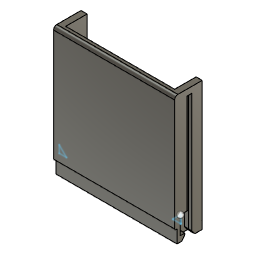
ExpansionCard (Autodesk Fusion 360 design; units mm, degrees)
Autodesk Fusion 360 part; units mm, degrees
sketch "Sketch1" plane through (0, 0, 0) normal (0, 0, 1) x (1, 0, 0)
ref_plane "WorkPlane1" through (0, 0, 0) normal (0, 0, 1) x (1, 0, 0)
sketch "Sketch2" plane through (0, 0, 0) normal (0, 0, 1) x (1, 0, 0)
  line L0 (-0.0018, 6.8149) -> (30, 6.8149)
  line L1 (30, 6.8149) -> (30, 0)
  line L2 (30, 0) -> (-0.0018, 0)
  line L3 (-0.0018, 0) -> (-0.0018, 6.8149)
  line L4 (14.9991, 3.4075) -> (25.7991, 3.4075)
  line L5 (14.9991, 3.4075) -> (4.1991, 3.4075)
  line L6 (14.9991, 4.3075) -> (4.6991, 4.3075)
  line L7 (14.9991, 4.3075) -> (25.2991, 4.3075)
  line L8 (14.9991, 2.5075) -> (4.6991, 2.5075)
  line L9 (14.9991, 2.5075) -> (25.2991, 2.5075)
  line L10 (14.9991, 4.3075) -> (25.2991, 4.3075)
  line L11 (14.9991, 4.3075) -> (4.6991, 4.3075)
  line L12 (25.7991, 3.8075) -> (25.7991, 3.4075)
  line L13 (4.1991, 3.0075) -> (4.1991, 3.4075)
  line L14 (4.1991, 3.8075) -> (4.1991, 3.4075)
  line L15 (25.7991, 3.4075) -> (25.7991, 3.0075)
  arc A0 (4.6991, 4.3075) -> (4.1991, 3.8075) centre (4.6991, 3.8075) ccw
  arc A1 (4.1991, 3.0075) -> (4.6991, 2.5075) centre (4.6991, 3.0075) ccw
  arc A2 (25.2991, 2.5075) -> (25.7991, 3.0075) centre (25.2991, 3.0075) ccw
  arc A3 (25.7991, 3.8075) -> (25.2991, 4.3075) centre (25.2991, 3.8075) ccw
  line L16 (14.9991, 3.4075) -> (14.9995, 3.4074)
  line L17 (15, 3.4075) -> (14.9995, 3.4074)
  dimension "d2" = 10.8
  dimension "d3" = 10.8
  dimension "d8" = 0.5
  constraint horizontal L0
  constraint vertical L1
  constraint horizontal L2
  constraint vertical L3
  constraint parallel L2 L4
  constraint parallel L4 L5
  constraint perpendicular L4 L12
  constraint perpendicular L5 L13
  constraint perpendicular L5 L14
  constraint parallel L5 L6
  constraint parallel L4 L7
  constraint tangent L14 A0
  constraint tangent L6 A0
  constraint parallel L5 L8
  constraint tangent L13 A1
  constraint tangent L8 A1
  constraint equal A0 A1
  constraint parallel L4 L9
  constraint tangent L9 A2
  constraint tangent L15 A2
  constraint equal A0 A2
  constraint tangent L12 A3
  constraint tangent L7 A3
  constraint equal A0 A3
  constraint parallel L4 L10
  constraint parallel L5 L11
  constraint coincident L4 L17.start
  measures "d2" distance of L4.start L4.end
  measures "d3" distance of L4.start L5.end
  measures "d8" radius of A0
other "Base Mesh Feature2"
sketch "Sketch4" plane through (0, 0, 0) normal (1, 0, 0) x (0, 1, 0)
  line L0 (6.8002, -0.0004) -> (6.8002, 32)
  line L1 (6.8002, 32) -> (0.8415, 32)
  line L2 (6.8002, -0.0004) -> (-0.2407, -0.0004)
  line L3 (-0.0066, 3.4989) -> (-0.0585, 31.0983)
  line L4 (4.9902, -0.0004) -> (4.2999, 0.9325)
  line L5 (4.2999, 0.9325) -> (4.25, 0.9325)
  line L6 (4.25, 0.9325) -> (4.25, 4.0597)
  line L7 (4.25, 4.0597) -> (2.5001, 4.0597)
  line L8 (2.5001, 1.39) -> (2.5001, 0.9325)
  line L9 (2.5001, 0.9325) -> (2.4506, 0.9325)
  line L10 (2.4506, 0.9325) -> (1.7589, -0.0004)
  line L11 (2.5001, 1.39) -> (1.4001, 1.39)
  line L12 (1.4001, 1.39) -> (1.4001, 5.86)
  line L13 (1.4001, 5.86) -> (3.0784, 5.86)
  line L14 (3.0784, 5.86) -> (3.0784, 30.5)
  line L15 (3.0784, 30.5) -> (4.25, 30.5)
  line L16 (4.25, 30.5) -> (4.25, 4.0597)
  line L17 (0.5999, -0.0004) -> (0.5999, 3.2)
  line L18 (0.5999, 3.2) -> (0.294, 3.1994)
  arc A0 (0.8415, 32) -> (-0.0585, 31.0983) centre (0.8415, 31.1) ccw
  arc A1 (-0.0066, 3.4989) -> (0.294, 3.1994) centre (0.2934, 3.4994) ccw
  line L19 (2.5001, 4.0597) -> (1.4001, 4.0597)
  dimension "d9" = 0.9
  dimension "d10" = 0.3
  constraint vertical L0
  constraint perpendicular L0 L1
  constraint perpendicular L0 L2
  constraint coincident L2 L4.start
  constraint parallel L2 L5
  constraint perpendicular L5 L6
  constraint perpendicular L6 L7
  constraint perpendicular L7 L8
  constraint perpendicular L8 L9
  constraint coincident L2 L10.end
  constraint perpendicular L8 L11
  constraint perpendicular L11 L12
  constraint perpendicular L12 L13
  constraint perpendicular L13 L14
  constraint perpendicular L14 L15
  constraint coincident L2 L17.start
  constraint perpendicular L2 L17
  constraint perpendicular L3 L18
  constraint tangent L1 A0
  constraint tangent L3 A0
  constraint tangent L18 A1
  constraint tangent L3 A1
  constraint coincident L12 L19.end
  constraint perpendicular L12 L19
  measures "d9" radius of A0
  measures "d10" radius of A1
ref_plane "WorkPlane2" through (14.9991, 3.4075, 32) normal (0, 0, 1) x (1, 0, 0)
sketch "Sketch5" plane through (14.9991, 3.4075, 32) normal (0, 0, 1) x (1, 0, 0)
  line L0 (-14.9991, 3.3927) -> (-14.9991, -3.4075)
  line L1 (-14.9991, -3.4075) -> (15.0009, -3.4075)
  line L2 (15.0009, -3.4075) -> (15.0009, 3.4075)
  line L3 (13.5009, 3.3927) -> (13.5009, 3.4067)
  line L4 (13.5009, 3.3927) -> (13.5009, -1.9074)
  line L5 (13.5009, -1.9074) -> (-13.4991, -1.9074)
  line L6 (-13.4991, -1.9074) -> (-13.5017, 3.3934)
  line L7 (15.0009, 3.4075) -> (13.5009, 3.4067)
  line L8 (-13.5017, 3.3934) -> (-14.9991, 3.3927)
  point P0 (-14.9991, 3.3927)
  point P1 (-14.9991, -3.4075)
  point P2 (15.0009, -3.4075)
  point P3 (15.0009, 3.4075)
  constraint coincident P0 L0.start
  constraint coincident P1 L0.end
  constraint coincident P2 L1.end
  constraint coincident P3 L2.end
  constraint perpendicular L3 L7
  constraint perpendicular L1 L4
  constraint perpendicular L4 L5
  constraint coincident L6.end L7
  constraint perpendicular L6 L7
  constraint collinear L7 L8
other "Modify1"
extrude "Extrude1" add sketch "Sketch5" against normal blind 32
extrude "Extrude2" add sketch "Sketch2" along normal blind 2
other "Modify2"
sketch "Side Slats" plane through (0, 0, 0) normal (0, 0, 1) x (1, 0, 0)
  line L0 (29.9999, 3.0777) -> (29.19, 3.93)
  line L1 (29.19, 3.93) -> (29.19, 4.25)
  line L2 (29.19, 4.25) -> (30, 4.25)
  line L3 (-0.0001, 3.0776) -> (0.81, 3.93)
  line L4 (0.81, 3.93) -> (0.81, 4.25)
  line L5 (0.81, 4.25) -> (0, 4.25)
  line L6 (-0.0001, 3.0776) -> (-0.201, 2.8662)
  line L7 (-0.201, 2.8662) -> (-0.2009, 4.25)
  line L8 (0, 4.25) -> (-0.2009, 4.25)
  line L9 (30, 4.25) -> (30.168, 4.25)
  line L10 (29.9999, 3.0777) -> (30.168, 2.9008)
  line L11 (30.168, 2.9008) -> (30.168, 4.25)
  constraint vertical L1
  constraint perpendicular L1 L2
  constraint vertical L4
  constraint perpendicular L4 L5
  constraint parallel L3 L6
  constraint perpendicular L7 L8
  constraint parallel L0 L10
  constraint perpendicular L9 L11
extrude "Extrude16" cut sketch "Side Slats" along normal blind 30.5
sketch "Sketch7" plane through (0, 0, 0) normal (1, 0, 0) x (0, 1, 0)
extrude "Extrude4" cut sketch "Sketch4" along normal blind 1.8 contours L2 L4 L5 L6 L7 L8 L9 L10 L11 L12 L19
extrude "Extrude5" cut sketch "Sketch4" against normal blind 1.2 contours L2 L4 L5 L6 L7 L8 L9 L10 L11 L12 L19
ref_plane "WorkPlane3" through (30, 0, 0) normal (1, 0, 0) x (0, 1, 0)
sketch "Sketch8" plane through (30, 0, 0) normal (1, 0, 0) x (0, 1, 0)
  line L0 (1.76, 0) -> (2.4501, 0.9324)
  line L1 (2.4501, 0.9324) -> (2.5001, 0.9324)
  line L2 (2.5001, 0.9324) -> (2.5001, 1.3897)
  line L3 (2.5001, 4.0595) -> (4.25, 4.0602)
  line L4 (4.25, 4.0602) -> (4.25, 0.9324)
  line L5 (4.25, 0.9324) -> (4.3, 0.9324)
  line L6 (4.3, 0.9324) -> (4.9902, -0.0001)
  line L7 (4.9902, -0.0001) -> (1.76, 0)
  line L8 (2.5001, 1.3897) -> (1.4001, 1.3897)
  line L9 (1.4001, 1.3897) -> (1.4001, 4.06)
  line L10 (1.4001, 4.06) -> (2.5001, 4.0595)
  constraint horizontal L1
  constraint perpendicular L1 L2
  constraint perpendicular L1 L4
  constraint perpendicular L4 L5
  constraint perpendicular L2 L8
  constraint perpendicular L8 L9
extrude "Extrude6" cut sketch "Sketch8" against normal blind 1.8
ref_plane "WorkPlane4" through (0, 0, 1.5) normal (0, 0, 1) x (1, 0, 0)
sketch "Sketch9" plane through (0, 0, 1.5) normal (0, 0, 1) x (1, 0, 0)
  line L0 (1.5, 5.3) -> (2.5, 5.3)
  line L1 (2.5, 5.3) -> (2.5, 1.5)
  line L2 (2.5, 1.5) -> (1.5, 1.5)
  line L3 (28.5, 5.3) -> (27.5, 5.3)
  line L4 (27.5, 5.3) -> (27.5, 1.5001)
  line L5 (27.5, 1.5001) -> (28.5, 1.5001)
  line L6 (1.6305, 5.3) -> (1.4386, 5.3)
  line L7 (1.4386, 5.3) -> (1.4386, 1.5)
  line L8 (1.4386, 1.5) -> (1.5958, 1.5)
  line L9 (28.4487, 5.3) -> (28.5452, 5.3)
  line L10 (28.5452, 5.3) -> (28.5453, 1.5001)
  line L11 (28.4238, 1.5001) -> (28.5453, 1.5001)
  constraint horizontal L0
  constraint perpendicular L0 L1
  constraint perpendicular L1 L2
  constraint horizontal L3
  constraint perpendicular L3 L4
  constraint perpendicular L4 L5
  constraint coincident L0 L6.start
  constraint parallel L0 L6
  constraint perpendicular L2 L7
  constraint coincident L2 L8.end
  constraint parallel L2 L8
  constraint coincident L3 L9.start
  constraint perpendicular L9 L10
  constraint coincident L5 L11.start
  constraint perpendicular L10 L11
extrude "Extrude7" add sketch "Sketch9" along normal blind 4 contours L0 L1 L2 L6 L7 L8
extrude "Extrude8" add sketch "Sketch9" along normal blind 4 contours L3 L4 L5 L9 L10 L11
ref_plane "WorkPlane5" through (0, 6, 0) normal (0, 1, 0) x (0, 0, 1)
sketch "Sketch10" plane through (0, 6, 0) normal (0, 1, 0) x (1, 0, 0)
  line L0 (2.5, -4.5) -> (1.5001, -5.5)
  line L1 (1.5001, -5.5) -> (2.5, -5.5)
  line L2 (2.5, -5.5) -> (2.5, -4.5)
  line L3 (28.5, -5.5) -> (27.5, -5.5)
  line L4 (27.5, -5.5) -> (27.5, -4.5)
  line L5 (27.5, -4.5) -> (28.5, -5.5)
  constraint horizontal L1
  constraint perpendicular L1 L2
  constraint perpendicular L2 L3
  constraint perpendicular L3 L4
extrude "Extrude9" cut sketch "Sketch10" against normal blind 4.5
extrude "Extrude10" cut sketch "Sketch8" against normal blind 1.8
extrude "Extrude11" cut sketch "Sketch4" along normal blind 1.8 contours L2 L4 L5 L6 L7 L8 L9 L10 L11 L12 L19
sketch "Sketch11" plane through (30, 0, 0) normal (1, 0, 0) x (0, 1, 0)
  line L0 (1.76, 0) -> (2.4501, 0.9324)
  line L1 (2.4501, 0.9324) -> (2.5001, 0.9324)
  line L2 (2.5001, 0.9324) -> (2.5001, 1.3897)
  line L3 (2.5001, 1.3897) -> (1.4001, 1.3897)
  line L4 (1.4001, 1.3897) -> (1.4001, 4.06)
  line L5 (1.4001, 4.06) -> (2.5001, 4.0595)
  line L6 (2.5001, 4.0595) -> (3.0776, 4.0597)
  line L7 (6.8149, 32) -> (0, 32)
  line L8 (0, 32) -> (0, 0)
  line L9 (4.9901, 0) -> (6.8149, 0)
  line L10 (0.6001, 0) -> (0.012, 0)
  line L11 (0.012, 3.1995) -> (0.6001, 3.1995)
  line L12 (0.6001, 3.1995) -> (0.6001, 0)
  line L13 (0.0679, 0) -> (-0.3097, 0)
  line L14 (-0.3097, 0) -> (-0.3097, 3.1995)
  line L15 (0.0854, 3.1995) -> (-0.3097, 3.1995)
  line L16 (0, 3.5529) -> (0, 3.1995)
  line L17 (0.6001, 3.1408) -> (0.6001, 3.6309)
  line L18 (0.6001, 3.6309) -> (0, 3.6309)
  line L19 (0, 3.5218) -> (0, 3.6309)
  line L20 (3.0776, 4.0597) -> (3.0776, 30.5)
  line L21 (3.0776, 30.5) -> (4.25, 30.5)
  line L22 (4.25, 30.5) -> (4.25, 0.9324)
  line L23 (4.25, 0.9324) -> (4.3, 0.9324)
  line L24 (4.3, 0.9324) -> (4.9901, 0)
  line L25 (6.8149, 0) -> (6.8149, 2)
  line L26 (6.8149, 2) -> (6.8149, 32)
  line L27 (0, 0) -> (1.76, 0)
  constraint horizontal L10
  constraint horizontal L11
  constraint vertical L12
  constraint coincident L9 L10.start
  constraint coincident L10 L13.start
  constraint perpendicular L13 L14
  constraint coincident L11 L15.start
  constraint perpendicular L14 L15
  constraint coincident L8 L16.start
  constraint coincident L15 L16.end
  constraint coincident L8 L16.end
  constraint perpendicular L15 L16
  constraint coincident L12 L17.start
  constraint perpendicular L11 L17
  constraint coincident L8 L18.end
  constraint perpendicular L8 L18
  constraint coincident L16 L19.start
extrude "Extrude12" cut sketch "Sketch11" against normal through all contours L8 L10 L11 L12 L13 L15 L17 L27 | L8 L13 L14 L15
sketch "Sketch12" plane through (30, 0, 0) normal (1, 0, 0) x (0, 1, 0)
  line L0 (0.6001, 3.1995) -> (0.6001, 0)
  line L1 (0.6001, 0) -> (1.76, 0)
  line L2 (1.76, 0) -> (2.4501, 0.9324)
  line L3 (2.4501, 0.9324) -> (2.5001, 0.9324)
  line L4 (2.5001, 0.9324) -> (2.5001, 1.3897)
  line L5 (2.5001, 1.3897) -> (1.4001, 1.3897)
  line L6 (1.4001, 1.3897) -> (1.4001, 4.06)
  line L7 (1.4001, 4.06) -> (2.5001, 4.0595)
  line L8 (2.5001, 4.0595) -> (3.0776, 4.0597)
  line L9 (6.8149, 32) -> (0, 32)
  line L10 (0, 32) -> (0, 3.1995)
  line L11 (0, 3.1995) -> (0.6001, 3.1995)
  line L12 (0, 3.4998) -> (0.716, 3.4998)
  line L13 (0.6001, 3.1995) -> (0.6001, 3.4998)
  line L14 (0, 3.4998) -> (0, 3.4995)
  line L15 (0.6001, 3.1995) -> (0.3, 3.1995)
  arc A0 (0, 3.4995) -> (0.3, 3.1995) centre (0.3, 3.4995) ccw
  line L16 (3.0776, 4.0597) -> (3.0776, 30.5)
  line L17 (3.0776, 30.5) -> (4.25, 30.5)
  line L18 (4.25, 30.5) -> (4.25, 0.9324)
  line L19 (4.25, 0.9324) -> (4.3, 0.9324)
  line L20 (4.3, 0.9324) -> (4.9901, 0)
  line L21 (4.9901, 0) -> (6.8149, 0)
  line L22 (6.8149, 0) -> (6.8149, 2)
  line L23 (6.8149, 2) -> (6.8149, 32)
  dimension "d37" = 0.3
  constraint coincident L10 L12.start
  constraint perpendicular L10 L12
  constraint coincident L0.start L11.end
  constraint coincident L12 L13.end
  constraint perpendicular L12 L13
  constraint tangent L15 A0
  constraint tangent L14 A0
  measures "d37" radius of A0
extrude "Extrude13" cut sketch "Sketch12" against normal through all contours L10 L11 A0
sketch "Sketch13" plane through (0, 0, 0) normal (0, 0, -1) x (1, 0, 0)
  line L0 (25.7991, -3.0075) -> (25.7991, -3.8075)
  arc A0 (25.2991, -4.3075) -> (25.7991, -3.8075) centre (25.2991, -3.8075) ccw
  line L1 (25.2991, -4.3075) -> (4.6991, -4.3075)
  arc A1 (4.1991, -3.8075) -> (4.6991, -4.3075) centre (4.6991, -3.8075) ccw
  line L2 (4.1991, -3.8075) -> (4.1991, -3.0075)
  arc A2 (4.6991, -2.5075) -> (4.1991, -3.0075) centre (4.6991, -3.0075) ccw
  line L3 (4.6991, -2.5075) -> (25.2991, -2.5075)
  arc A3 (25.7991, -3.0075) -> (25.2991, -2.5075) centre (25.2991, -3.0075) ccw
  line L4 (30, -0.6001) -> (-0.0018, -0.6001)
  line L5 (-0.0018, -0.6001) -> (-0.0018, -1.7592)
  line L6 (-0.0018, -1.7592) -> (1.8, -1.7592)
  line L7 (1.8, -1.7592) -> (1.8, -4.9899)
  line L8 (1.8, -4.9899) -> (-0.0018, -4.9899)
  line L9 (-0.0018, -4.9899) -> (-0.0018, -6.8149)
  line L10 (-0.0018, -6.8149) -> (30, -6.8149)
  line L11 (30, -6.8149) -> (30, -4.9901)
  line L12 (30, -4.9901) -> (28.2, -4.9901)
  line L13 (28.2, -4.9901) -> (28.2, -1.76)
  line L14 (28.2, -1.76) -> (30, -1.76)
  line L15 (30, -1.76) -> (30, -0.6001)
  line L16 (14.6109, -2.2) -> (17.9456, -2.2)
  line L17 (19.2456, -3.5) -> (19.2456, -3.5306)
  line L18 (17.9456, -4.8306) -> (14.6109, -4.8306)
  line L19 (14.6109, -2.2) -> (12.0539, -2.2)
  line L20 (10.7539, -3.5) -> (10.7539, -3.5306)
  line L21 (12.0539, -4.8306) -> (14.6109, -4.8306)
  arc A4 (12.0539, -2.2) -> (10.7539, -3.5) centre (12.0539, -3.5) ccw
  arc A5 (10.7539, -3.5306) -> (12.0539, -4.8306) centre (12.0539, -3.5306) ccw
  arc A6 (19.2456, -3.5) -> (17.9456, -2.2) centre (17.9456, -3.5) ccw
  arc A7 (17.9456, -4.8306) -> (19.2456, -3.5306) centre (17.9456, -3.5306) ccw
  dimension "d39" = 1.3
  dimension "d40" = 1.3
  dimension "d41" = 1.3
  dimension "d42" = 1.3
  constraint horizontal L16
  constraint vertical L17
  constraint horizontal L18
  constraint horizontal L19
  constraint vertical L20
  constraint horizontal L21
  constraint tangent L20 A4
  constraint tangent L19 A4
  constraint tangent L20 A5
  constraint tangent L21 A5
  constraint tangent L16 A6
  constraint tangent L17 A6
  constraint tangent L17 A7
  constraint tangent L18 A7
  measures "d39" radius of A4
  measures "d40" radius of A5
  measures "d41" radius of A6
  measures "d42" radius of A7
extrude "Extrude14" add sketch "Sketch13" against normal blind 2 contours L0 A0 L1 L3 A3 L17 A6 A7 | L1 L3 L17 L20 A4 A5 A6 A7 | L1 A1 L2 A2 L3 L20 A4 A5
extrude "Extrude15" cut sketch "Sketch13" against normal through all contours L1 L3 L17 L20 A4 A5 A6 A7 | L3 L16 L19 A4 A6 | L1 L18 L21 A5 A7
sketch "Sketch14" plane through (30, 0, 0) normal (1, 0, 0) x (0, 1, 0)
  arc A0 (0, 3.4995) -> (0.3, 3.1995) centre (0.3, 3.4995) ccw
  line L0 (0.3, 3.1995) -> (0.6001, 3.1995)
  line L1 (0.6001, 3.1995) -> (0.6001, 0)
  line L2 (0.6001, 0) -> (1.76, 0)
  line L3 (1.76, 0) -> (2.4501, 0.9324)
  line L4 (2.4501, 0.9324) -> (2.5001, 0.9324)
  line L5 (2.5001, 0.9324) -> (2.5001, 1.3897)
  line L6 (2.5001, 1.3897) -> (1.4001, 1.3897)
  line L7 (1.4001, 1.3897) -> (1.4001, 4.06)
  line L8 (1.4001, 4.06) -> (2.5001, 4.0595)
  line L9 (2.5001, 4.0595) -> (3.0776, 4.0597)
  line L10 (3.0776, 4.0597) -> (3.0776, 30.5)
  line L11 (3.0776, 30.5) -> (4.25, 30.5)
  line L12 (4.25, 30.5) -> (4.25, 0.9324)
  line L13 (4.25, 0.9324) -> (4.3, 0.9324)
  line L14 (4.3, 0.9324) -> (4.9901, 0)
  line L15 (4.9901, 0) -> (6.8149, 0)
  line L16 (6.8149, 0) -> (6.8149, 2)
  line L17 (6.8149, 2) -> (6.8149, 32)
  line L18 (6.8149, 32) -> (0, 32)
  line L19 (0, 32) -> (0, 3.4995)
  line L20 (0.8001, 32) -> (0.8, 32)
  line L21 (0, 31.2) -> (0, 31.2001)
  line L22 (0, 31.2001) -> (0.8001, 31.2001)
  line L23 (0.8001, 31.2001) -> (0.8001, 32)
  arc A1 (0.8, 32) -> (0, 31.2) centre (0.8, 31.2) ccw
  dimension "d48" = 0.8
  constraint horizontal L20
  constraint vertical L21
  constraint horizontal L22
  constraint vertical L23
  constraint coincident L19 L21.end
  constraint coincident L18 L20.start
  constraint tangent L21 A1
  constraint tangent L20 A1
  measures "d48" radius of A1
extrude "Extrude17" cut sketch "Sketch14" against normal through all contours L18 L19 A1
ref_plane "WorkPlane6" through (0, 1.4, 0) normal (0, 1, 0) x (0, 0, 1)
sketch "Sketch15" plane through (0, 1.4, 0) normal (0, 1, 0) x (1, 0, 0)
  line L0 (1.8, -4.0597) -> (0, -5.8599)
  line L1 (0, -5.8599) -> (0, -4.0597)
  line L2 (0, -4.0597) -> (1.8, -4.0597)
  line L3 (28.2005, -4.0596) -> (30, -5.8599)
  line L4 (30.0677, -4.0596) -> (30.0677, -5.9277)
  line L5 (29.9608, -5.8208) -> (30.0677, -5.9277)
  line L6 (30.0677, -4.0596) -> (30.0677, -3.9862)
  line L7 (30.0677, -3.9862) -> (28.2005, -3.9862)
  line L8 (28.2005, -4.0596) -> (28.2005, -3.9862)
  constraint vertical L1
  constraint perpendicular L1 L2
  constraint coincident L3 L5.start
  constraint parallel L3 L5
  constraint perpendicular L6 L7
  constraint perpendicular L7 L8
extrude "Extrude18" cut sketch "Sketch15" along normal blind 2.85 contours L0 L1 L2
extrude "Extrude19" cut sketch "Sketch15" along normal blind 2.85 contours L3 L4 L5 L6 L7 L8
